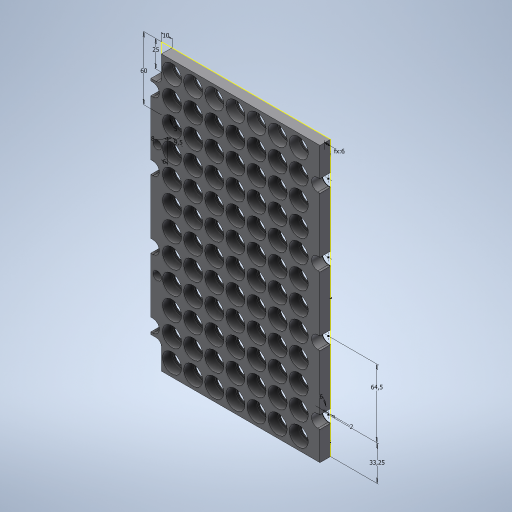
# Autodesk Inventor part: Platte1
Saved by Autodesk Inventor 2024 (Build 280153000, 153)
## iProperties
Created: 2025-03-19
Part Number: Platte1
Material: Generisch
Document SubType Name: Modeling
Designer: David Lill
Density: 1 g/cm^3
Appearance: Vorgabe
Author: David Lill
Autodesk Inventor part; units mm, degrees
ref_plane "YZ Plane" through (0, 0, 0) normal (1, 0, 0) x (0, 1, 0)
ref_plane "XZ Plane" through (0, 0, 0) normal (0, 1, 0) x (-1, 0, 0)
ref_plane "XY Plane" through (0, 0, 0) normal (0, 0, 1) x (1, 0, 0)
sketch "Skizze1" plane through (0, 0, 0) normal (0, 1, 0) x (-1, 0, 0)
  line L0 (160, 0) -> (0, 0)
  line L1 (0, 0) -> (0, -260)
  line L2 (0, -260) -> (160, -260)
  line L3 (160, -260) -> (160, 0)
  circle A0 centre (140, -11.75) radius 9
  circle A1 centre (140, -54.75) radius 9
  circle A2 centre (140, -97.75) radius 9
  circle A3 centre (140, -140.75) radius 9
  circle A4 centre (140, -183.75) radius 9
  circle A5 centre (140, -226.75) radius 9
  circle A6 centre (120, -11.75) radius 9
  circle A7 centre (120, -54.75) radius 9
  circle A8 centre (120, -97.75) radius 9
  circle A9 centre (120, -140.75) radius 9
  circle A10 centre (120, -183.75) radius 9
  circle A11 centre (120, -226.75) radius 9
  circle A12 centre (100, -11.75) radius 9
  circle A13 centre (100, -54.75) radius 9
  circle A14 centre (100, -97.75) radius 9
  circle A15 centre (100, -140.75) radius 9
  circle A16 centre (100, -183.75) radius 9
  circle A17 centre (100, -226.75) radius 9
  circle A18 centre (80, -11.75) radius 9
  circle A19 centre (80, -54.75) radius 9
  circle A20 centre (80, -97.75) radius 9
  circle A21 centre (80, -140.75) radius 9
  circle A22 centre (80, -183.75) radius 9
  circle A23 centre (80, -226.75) radius 9
  circle A24 centre (60, -11.75) radius 9
  circle A25 centre (60, -54.75) radius 9
  circle A26 centre (60, -97.75) radius 9
  circle A27 centre (60, -140.75) radius 9
  circle A28 centre (60, -183.75) radius 9
  circle A29 centre (60, -226.75) radius 9
  circle A30 centre (40, -11.75) radius 9
  circle A31 centre (40, -54.75) radius 9
  circle A32 centre (40, -97.75) radius 9
  circle A33 centre (40, -140.75) radius 9
  circle A34 centre (40, -183.75) radius 9
  circle A35 centre (40, -226.75) radius 9
  circle A36 centre (20, -11.75) radius 9
  circle A37 centre (20, -54.75) radius 9
  circle A38 centre (20, -97.75) radius 9
  circle A39 centre (20, -140.75) radius 9
  circle A40 centre (20, -183.75) radius 9
  circle A41 centre (20, -226.75) radius 9
  circle A42 centre (140, -33.25) radius 9
  circle A43 centre (120, -33.25) radius 9
  circle A44 centre (100, -33.25) radius 9
  circle A45 centre (80, -33.25) radius 9
  circle A46 centre (60, -33.25) radius 9
  circle A47 centre (40, -33.25) radius 9
  circle A48 centre (20, -33.25) radius 9
  circle A49 centre (140, -76.25) radius 9
  circle A50 centre (120, -76.25) radius 9
  circle A51 centre (100, -76.25) radius 9
  circle A52 centre (80, -76.25) radius 9
  circle A53 centre (60, -76.25) radius 9
  circle A54 centre (40, -76.25) radius 9
  circle A55 centre (20, -76.25) radius 9
  circle A56 centre (140, -119.25) radius 9
  circle A57 centre (120, -119.25) radius 9
  circle A58 centre (100, -119.25) radius 9
  circle A59 centre (80, -119.25) radius 9
  circle A60 centre (60, -119.25) radius 9
  circle A61 centre (40, -119.25) radius 9
  circle A62 centre (20, -119.25) radius 9
  circle A63 centre (140, -162.25) radius 9
  circle A64 centre (120, -162.25) radius 9
  circle A65 centre (100, -162.25) radius 9
  circle A66 centre (80, -162.25) radius 9
  circle A67 centre (60, -162.25) radius 9
  circle A68 centre (40, -162.25) radius 9
  circle A69 centre (20, -162.25) radius 9
  circle A70 centre (140, -205.25) radius 9
  circle A71 centre (120, -205.25) radius 9
  circle A72 centre (100, -205.25) radius 9
  circle A73 centre (80, -205.25) radius 9
  circle A74 centre (60, -205.25) radius 9
  circle A75 centre (40, -205.25) radius 9
  circle A76 centre (20, -205.25) radius 9
  circle A77 centre (140, -248.25) radius 9
  circle A78 centre (120, -248.25) radius 9
  circle A79 centre (100, -248.25) radius 9
  circle A80 centre (80, -248.25) radius 9
  circle A81 centre (60, -248.25) radius 9
  circle A82 centre (40, -248.25) radius 9
  circle A83 centre (20, -248.25) radius 9
  line L4 (-20, 0) -> (-187, 0)
  line L5 (-207, 0) -> (-374, 0)
  circle A84 centre (140, -11.75) radius 7.5
  line L6 (155.379, -44.5989) -> (146.379, -44.5989)
  line L7 (157, -62) -> (150, -62)
  line L8 (150, -62) -> (150, -69)
  line L9 (150, -69) -> (157, -69)
  line L10 (157, -69) -> (157, -62)
  line L11 (160, -130) -> (0, -130) construction
  line L12 (157, -198) -> (150, -198)
  line L13 (150, -198) -> (150, -191)
  line L14 (150, -191) -> (157, -191)
  line L15 (157, -191) -> (157, -198)
  point P0 (80, 0)
  point P1 (153.5, -62)
  point P2 (157, -65.5)
  dimension "d0" = 160
  dimension "d1" = 260
  dimension "d4" = 18
  dimension "d7" = 43
  dimension "d10" = 20
  dimension "d16" = 21.5
  dimension "d21" = 20
  dimension "d24" = 43
  dimension "d69" = 15
  dimension "d80" = 0
  dimension "d127" = 10.75
  dimension "d129" = 7
  dimension "d130" = 7
  dimension "d132" = 3
  dimension "d134" = 10.75
  constraints: 85 centre point, 32 end point, 14 coincident, 6 horizontal, 5 midpoint, 4 parallel, 4 symmetric about line, 2 horizontal alignment, 2 perpendicular, 2 vertical, 1 equal radius, 1 vertical alignment, 164 other
  measures "d0" distance of L0.start L0.end
  measures "d1" distance of L2.end L0.start
  measures "d4" diameter of A0
  measures "d7" distance of A0.centre A1.centre
  measures "d10" distance of A0.centre A6.centre
  measures "d16" distance of A42.centre A0.centre
  measures "d21" distance of A42.centre A43.centre
  measures "d24" distance of A42.centre A49.centre
  measures "d69" diameter of A84
  measures "d80" horizontal distance of A0.centre A42.centre
  measures "d127" vertical distance of L11.start point (140, -119.25)
  measures "d129" distance of L9.end L8.end
  measures "d130" distance of L8.end L7.end
  measures "d132" distance between parallel lines of L3 L10
  measures "d134" vertical distance of point (140, -76.25) point (157, -65.5)
extrude "Extrusion1" add sketch "Skizze1" along normal blind 10 contours L3 L2 L1 L0 | A0 | A1 | A2 | A3 | A4 | A5 | A6 | A7 | A8 | A9 | A10 | A11 | A12 | A13 | A14 | A15 | A16 | A17 | A18 | A19 | A20 | A21 | A22 | A23 | A24 | A25 | A26 | A27 | A28 | A29 | A30 | A31 | A32 | A33 | A34 | A35 | A36 | A37 | A38 | A39 | A40 | A41 | A42 | A43 | A44 | A45 | A46 | A47 | A48 | A49 | A50 | A51 | A52 | A53 | A54 | A55 | A56 | A57 | A58 | A59 | A60 | A61 | A62 | A63 | A64 | A65 | A66 | A67 | A68 | A69 | A70 | A71 | A72 | A73 | A74 | A75 | A76 | A77 | A78 | A79 | A80 | A81 | A82 | A83 | A84 | L10 L9 L8 L7 | L12 L13 L14 L15
hole "Bohrung1" at (-140, 0, -11.75) at (-140, 0, -33.25) at (-140, 0, -54.75) at (-140, 0, -76.25) at (-140, 0, -97.75) at (-140, 0, -119.25) at (-140, 0, -140.75) at (-140, 0, -162.25) at (-140, 0, -183.75) at (-140, 0, -205.25) at (-140, 0, -226.75) at (-140, 0, -248.25) direction (0, 1, 0) diameter 15 end through all counterbore diameter 18 counterbore depth 9
pattern_linear "Rechteckige Anordnung1" count 7 spacing 20 along (1, 0, 0) of "Bohrung1"
sketch "Skizze2" plane through (0, 10, 0) normal (0, 1, 0) x (1, 0, 0)
  circle A0 centre (-20, 226.75) radius 9 projected
  circle A1 centre (-20, 248.25) radius 9 projected
  circle A2 centre (-20, 205.25) radius 9 projected
  circle A3 centre (-20, 162.25) radius 9 projected
  circle A4 centre (-20, 119.25) radius 9 projected
  circle A5 centre (-20, 76.25) radius 9
  circle A6 centre (-20, 33.25) radius 9 projected
  circle A7 centre (-20, 11.75) radius 9 projected
  circle A8 centre (-20, 54.75) radius 9 projected
  circle A9 centre (-20, 97.75) radius 9 projected
  circle A10 centre (-20, 140.75) radius 9 projected
  circle A11 centre (-20, 183.75) radius 9 projected
  circle A12 centre (-40, 226.75) radius 9 projected
  circle A13 centre (-40, 248.25) radius 9 projected
  circle A14 centre (-40, 205.25) radius 9 projected
  circle A15 centre (-40, 162.25) radius 9 projected
  circle A16 centre (-40, 119.25) radius 9 projected
  circle A17 centre (-40, 76.25) radius 9 projected
  circle A18 centre (-40, 33.25) radius 9 projected
  circle A19 centre (-40, 11.75) radius 9 projected
  circle A20 centre (-40, 54.75) radius 9 projected
  circle A21 centre (-40, 97.75) radius 9 projected
  circle A22 centre (-40, 140.75) radius 9 projected
  circle A23 centre (-40, 183.75) radius 9 projected
  circle A24 centre (-60, 226.75) radius 9 projected
  circle A25 centre (-60, 248.25) radius 9 projected
  circle A26 centre (-60, 205.25) radius 9 projected
  circle A27 centre (-60, 162.25) radius 9 projected
  circle A28 centre (-60, 119.25) radius 9 projected
  circle A29 centre (-60, 76.25) radius 9 projected
  circle A30 centre (-60, 33.25) radius 9 projected
  circle A31 centre (-60, 11.75) radius 9 projected
  circle A32 centre (-60, 54.75) radius 9 projected
  circle A33 centre (-60, 97.75) radius 9 projected
  circle A34 centre (-60, 140.75) radius 9 projected
  circle A35 centre (-60, 183.75) radius 9 projected
  circle A36 centre (-80, 226.75) radius 9 projected
  circle A37 centre (-80, 248.25) radius 9 projected
  circle A38 centre (-80, 205.25) radius 9 projected
  circle A39 centre (-80, 162.25) radius 9 projected
  circle A40 centre (-80, 119.25) radius 9 projected
  circle A41 centre (-80, 76.25) radius 9 projected
  circle A42 centre (-80, 33.25) radius 9 projected
  circle A43 centre (-80, 11.75) radius 9 projected
  circle A44 centre (-80, 54.75) radius 9 projected
  circle A45 centre (-80, 97.75) radius 9 projected
  circle A46 centre (-80, 140.75) radius 9 projected
  circle A47 centre (-80, 183.75) radius 9 projected
  circle A48 centre (-100, 226.75) radius 9 projected
  circle A49 centre (-100, 248.25) radius 9 projected
  circle A50 centre (-100, 205.25) radius 9 projected
  circle A51 centre (-100, 162.25) radius 9 projected
  circle A52 centre (-100, 119.25) radius 9 projected
  circle A53 centre (-100, 76.25) radius 9 projected
  circle A54 centre (-100, 33.25) radius 9 projected
  circle A55 centre (-100, 11.75) radius 9 projected
  circle A56 centre (-100, 54.75) radius 9 projected
  circle A57 centre (-100, 97.75) radius 9 projected
  circle A58 centre (-100, 140.75) radius 9 projected
  circle A59 centre (-100, 183.75) radius 9 projected
  circle A60 centre (-120, 226.75) radius 9 projected
  circle A61 centre (-120, 248.25) radius 9 projected
  circle A62 centre (-120, 205.25) radius 9 projected
  circle A63 centre (-120, 162.25) radius 9 projected
  circle A64 centre (-120, 119.25) radius 9 projected
  circle A65 centre (-120, 76.25) radius 9 projected
  circle A66 centre (-120, 33.25) radius 9 projected
  circle A67 centre (-120, 11.75) radius 9 projected
  circle A68 centre (-120, 54.75) radius 9 projected
  circle A69 centre (-120, 97.75) radius 9 projected
  circle A70 centre (-120, 140.75) radius 9 projected
  circle A71 centre (-120, 183.75) radius 9 projected
  circle A72 centre (-140, 226.75) radius 9 projected
  circle A73 centre (-140, 183.75) radius 9 projected
  circle A74 centre (-140, 140.75) radius 9 projected
  circle A75 centre (-140, 97.75) radius 9 projected
  circle A76 centre (-140, 54.75) radius 9 projected
  circle A77 centre (-140, 11.75) radius 9 projected
  circle A78 centre (-140, 33.25) radius 9 projected
  circle A79 centre (-140, 76.25) radius 9 projected
  circle A80 centre (-140, 119.25) radius 9 projected
  circle A81 centre (-140, 162.25) radius 9 projected
  circle A82 centre (-140, 205.25) radius 9 projected
  circle A83 centre (-140, 248.25) radius 9 projected
  line L0 (0, 0) -> (0, 260) projected
  line L1 (-160, 0) -> (0, 0) projected
  line L2 (-160, 260) -> (-160, 0) projected
  line L3 (0, 260) -> (-160, 260) projected
  line L4 (-160, 0) -> (0, 0) projected
  line L5 (-150, 0) -> (-150, 55)
  arc A84 (-150, 55) -> (-155, 60) centre (-155, 55) ccw
  line L6 (-155, 60) -> (-160, 60)
  line L7 (-160, 260) -> (-160, 0) projected
  line L8 (-160, 0) -> (0, 0) projected
  line L9 (0, 0) -> (0, 260) projected
  line L10 (-160, 260) -> (-160, 0) projected
  line L11 (0, 260) -> (-160, 260) projected
  line L12 (-160, 25) -> (-155, 25)
  arc A85 (-150, 20) -> (-155, 25) centre (-155, 20) ccw
  line L13 (0, 130) -> (-160, 130)
  line L14 (-150, 260) -> (-150, 205)
  arc A86 (-155, 200) -> (-150, 205) centre (-155, 205) ccw
  line L15 (-155, 200) -> (-160, 200)
  line L16 (-160, 235) -> (-155, 235)
  arc A87 (-155, 235) -> (-150, 240) centre (-155, 240) ccw
  circle A88 centre (-20, 11.75) radius 9 projected
  line L17 (-143.0414, 85.25) -> (-151, 85.25)
  arc A89 (-151, 85.25) -> (-151, 67.25) centre (-151, 76.25) ccw
  line L18 (-151, 67.25) -> (-143.0414, 67.25)
  arc A90 (-143.0414, 85.25) -> (-143.0414, 67.25) centre (-140, 76.25) ccw
  line L19 (-143.0414, 174.75) -> (-151, 174.75)
  arc A91 (-151, 192.75) -> (-151, 174.75) centre (-151, 183.75) ccw
  line L20 (-151, 192.75) -> (-143.0414, 192.75)
  arc A92 (-143.0414, 192.75) -> (-143.0414, 174.75) centre (-140, 183.75) ccw
  circle A93 centre (-154, 76.25) radius 4
  circle A94 centre (-154, 183.75) radius 4
  line L21 (-80, 260) -> (-80, 0)
  line L22 (0, 232.75) -> (-2, 232.75)
  arc A95 (-2, 232.75) -> (-2, 220.75) centre (-2, 226.75) ccw
  line L23 (-2, 220.75) -> (0, 220.75)
  line L24 (0, 168.25) -> (-2, 168.25)
  arc A96 (-2, 168.25) -> (-2, 156.25) centre (-2, 162.25) ccw
  line L25 (-2, 156.25) -> (0, 156.25)
  line L26 (-160, 168.25) -> (-158, 168.25)
  arc A97 (-158, 156.25) -> (-158, 168.25) centre (-158, 162.25) ccw
  line L27 (-158, 156.25) -> (-160, 156.25)
  line L28 (0, 27.25) -> (-2, 27.25)
  arc A98 (-2, 39.25) -> (-2, 27.25) centre (-2, 33.25) ccw
  line L29 (-2, 39.25) -> (0, 39.25)
  line L30 (0, 91.75) -> (-2, 91.75)
  arc A99 (-2, 103.75) -> (-2, 91.75) centre (-2, 97.75) ccw
  line L31 (-2, 103.75) -> (0, 103.75)
  arc A100 (-158, 91.75) -> (-158, 103.75) centre (-158, 97.75) ccw
  line L32 (-160, 91.75) -> (-158, 91.75)
  line L33 (-158, 103.75) -> (-160, 103.75)
  line L34 (-16.9586, 20.75) -> (-9, 20.75)
  arc A101 (-9, 2.75) -> (-9, 20.75) centre (-9, 11.75) ccw
  line L35 (-9, 2.75) -> (-16.9586, 2.75)
  arc A102 (-16.9586, 2.75) -> (-16.9586, 20.75) centre (-20, 11.75) ccw
  circle A103 centre (-6, 11.75) radius 4
  arc A104 (-9, 239.25) -> (-9, 257.25) centre (-9, 248.25) ccw
  line L36 (-9, 257.25) -> (-16.9586, 257.25)
  arc A105 (-16.9586, 239.25) -> (-16.9586, 257.25) centre (-20, 248.25) ccw
  line L37 (-16.9586, 239.25) -> (-9, 239.25)
  circle A106 centre (-6, 248.25) radius 4
  circle A107 centre (-20, 76.25) radius 9
  circle A108 centre (-20, 76.25) radius 9 projected
  line L38 (-160, 232.75) -> (-158, 232.75)
  arc A109 (-158, 220.75) -> (-158, 232.75) centre (-158, 226.75) ccw
  line L39 (-158, 220.75) -> (-160, 220.75)
  arc A110 (-158, 27.25) -> (-158, 39.25) centre (-158, 33.25) ccw
  line L40 (-160, 27.25) -> (-158, 27.25)
  line L41 (-158, 39.25) -> (-160, 39.25)
  point P0 (-160, 60)
  point P1 (0, 130)
  point P2 (-150, 260)
  point P3 (-160, 200)
  point P4 (-160, 235)
  point P5 (-160, 25)
  point P6 (0, 27.25)
  point P7 (0, 39.25)
  point P8 (0, 103.75)
  dimension "d83" = 10
  dimension "d84" = 5
  dimension "d85" = 60
  dimension "d101" = 25
  dimension "d119" = 8
  dimension "d121" = 6
  dimension "d124" = 33.25
  dimension "d125" = 64.5
  dimension "d126" = 6
  dimension "d135" = 9.5
  dimension "d136" = 2
  dimension "d142" = 6
  constraints: 64 end point, 54 symmetric about line, 40 point on circle, 26 centre point, 14 tangent, 9 point on line, 6 coincident, 6 equal radius, 5 horizontal, 5 midpoint, 5 perpendicular, 4 horizontal alignment, 3 parallel, 2 concentric, 2 vertical, 2 vertical alignment, 14 other
  measures "d83" distance between parallel lines of L2 L5
  measures "d84" radius of A84
  measures "d85" distance between parallel lines of L6 L4
  measures "d101" distance between parallel lines of L4 L12
  measures "d119" diameter of A93
  measures "d121" distance from line of L2 A93.centre
  measures "d124" distance from line of L11 point (-2, 226.75)
  measures "d125" distance of point (-2, 226.75) point (-2, 162.25)
  measures "d126" radius of A95
  measures "d135" radius of A90
  measures "d136" distance from line of L0 point (-2, 226.75)
  measures "d142" distance from line of L9 A103.centre
extrude "Extrusion2" cut sketch "Skizze2" against normal blind 10 contours L14 A87 L16 L2 L3 | L12 A85 L5 L1 L2 | A93 | A94
extrude "Extrusion4" cut sketch "Skizze2" against normal up to surface (10 mm away) contours L0 L23 A95 L22 | L38 A109 L39 L2 | L0 L25 A96 L24 | L26 A97 L27 L2 | L0 L30 A99 L31 | L33 A100 L32 L2 | L0 L28 A98 L29 | L41 A110 L40 L2
equation "\"d16\" = 0.5 * d7"
equation "\"d21\" = d10"
equation "\"d24\" = d7"
